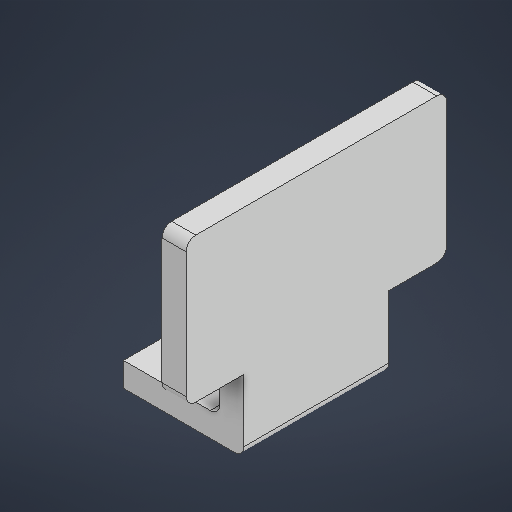
# Autodesk Inventor part: end plate
Saved by Autodesk Inventor 2027 (Build 310192000, 192)
## iProperties
Created: 2026-07-15
Part Number: end plate
Material: Generic
Document SubType Name: Modeling
Designer: ratik
Density: 1 g/cm^3
Appearance: Default
Author: ratik
Autodesk Inventor part; units mm, degrees
ref_plane "YZ Plane" through (0, 0, 0) normal (1, 0, 0) x (0, 1, 0)
ref_plane "XZ Plane" through (0, 0, 0) normal (0, 1, 0) x (-1, 0, 0)
ref_plane "XY Plane" through (0, 0, 0) normal (0, 0, 1) x (1, 0, 0)
sketch "Sketch1" plane through (0, 0, 0) normal (1, 0, 0) x (0, 1, 0)
  line L0 (32.6613, 26.3105) -> (-7.3387, 26.3105)
  line L1 (-7.3387, 26.3105) -> (-7.3387, -27.6895)
  line L2 (-7.3387, -27.6895) -> (32.6613, -27.6895)
  line L3 (32.6613, -27.6895) -> (32.6613, 26.3105)
  point P0 (0, 0)
  dimension "d0" = 40
  dimension "d1" = 54
  constraints: 8 end point, 2 parallel, 1 horizontal, 1 perpendicular
  measures "d0" distance of L0.start L0.end
  measures "d1" distance of L2.end L0.start
extrude "Extrusion1" add sketch "Sketch1" along normal blind 5
sketch "Sketch2" plane through (0, -7.3387, 26.3105) normal (0, 0, 1) x (1, 0, 0)
  line L0 (5, 0) -> (-20, 0)
  line L1 (-20, 0) -> (-20, -5)
  line L2 (-20, -5) -> (5, -5)
  line L3 (5, -5) -> (5, 0)
  point P0 (0, 7.3387)
  dimension "d4" = 5
  dimension "d5" = 25
  constraints: 8 end point, 2 parallel, 1 horizontal, 1 perpendicular
  measures "d4" distance of L2.end L0.start
  measures "d5" distance of L1.end L2.end
extrude "Extrusion2" add sketch "Sketch2" against normal blind 54
sketch "Sketch3" plane through (5, 0, 0) normal (1, 0, 0) x (0, 0, -1)
  line L0 (-26.3105, 32.6613) -> (-26.3105, -12.3387) projected
  line L1 (-26.3105, -12.3387) -> (-14.3105, -12.3387)
  line L2 (-14.3105, -12.3387) -> (-14.3105, 2.6613)
  line L3 (-14.3105, 2.6613) -> (-26.3105, 2.6613)
  line L4 (-26.3105, 2.6613) -> (-26.3105, -12.3387)
  line L5 (-26.3105, -12.3387) -> (27.6895, -12.3387) projected
  line L6 (27.6895, -12.3387) -> (15.6895, -12.3387)
  line L7 (15.6895, -12.3387) -> (15.6895, 2.6613)
  line L8 (15.6895, 2.6613) -> (27.6895, 2.6613)
  line L9 (27.6895, 2.6613) -> (27.6895, -12.3387)
  point P0 (0, 0)
  point P1 (15.6895, -12.3387)
  dimension "d8" = 12
  dimension "d9" = 12
  dimension "d10" = 15
  dimension "d11" = 15
  constraints: 16 end point, 4 parallel, 2 horizontal, 2 perpendicular
  measures "d8" distance of L2.end L3.end
  measures "d9" distance of L7.end L8.end
  measures "d10" distance of L6.end L7.end
  measures "d11" distance of L1.end L2.end
extrude "Extrusion3" cut sketch "Sketch3" against normal through all
fillet "Fillet1" radius 2 4 edges at (2.5, 2.6613, 26.3105) (2.5, 2.6613, -27.6895) (2.5, 32.6613, -27.6895) (2.5, 32.6613, 26.3105)
fillet "Fillet2" radius 2 1 edges at (0, -7.3387, -0.6895)
sketch "Sketch4" plane through (-20, -7.3387, 14.3105) normal (0, 1, 0) x (1, 0, 0)
  arc A0 (10.7679, 21.3) -> (4.5679, 21.3) centre (7.6679, 21.3) ccw
  arc A1 (4.5679, 8.9679) -> (10.7679, 8.9679) centre (7.6679, 8.9679) ccw
  line L0 (10.7679, 21.3) -> (10.7679, 8.9679)
  line L1 (4.5679, 21.3) -> (4.5679, 8.9679)
  line L2 (18, 30) -> (0, 30) projected
  point P0 (20, 14.3105)
  dimension "d16" = 6.2
  dimension "d17" = 6.2
  dimension "d18" = 8.7
  constraints: 4 end point, 4 point on circle, 2 centre point, 1 parallel, 1 tangent
  measures "d16" diameter of A0
  measures "d17" diameter of A1
  measures "d18" distance from line of L2 A0.centre
extrude "Extrusion4" cut sketch "Sketch4" against normal through all
fillet "Fillet3" radius 2 1 edges at (5, -12.3387, -0.6895)
body "Solid1"
